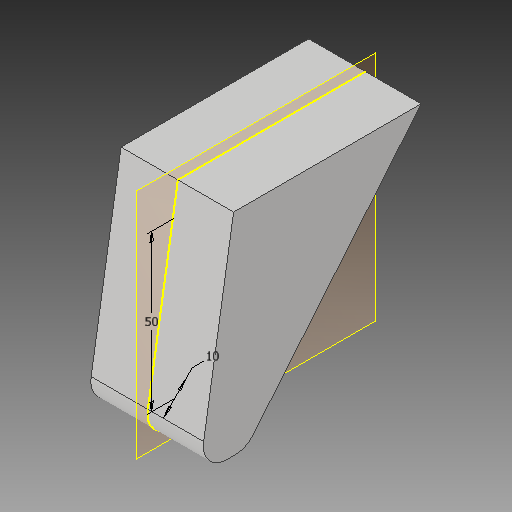
# Autodesk Inventor part: Part_MetalLeg
Saved by Autodesk Inventor 2019 (Build 230136000, 136)
## iProperties
Created: 2019-04-26
Part Number: Part_MetalLeg
Material: 일반
Document SubType Name: Modeling
Designer: hinmo
Density: 1 g/cm^3
Appearance: 기본값
Author: hinmo
Autodesk Inventor part; units mm, degrees
ref_plane "YZ Plane" through (0, 0, 0) normal (1, 0, 0) x (0, 1, 0)
ref_plane "XZ Plane" through (0, 0, 0) normal (0, 1, 0) x (-1, 0, 0)
ref_plane "XY Plane" through (0, 0, 0) normal (0, 0, 1) x (1, 0, 0)
sketch "스케치1" plane through (0, 0, 0) normal (1, 0, 0) x (0, 1, 0)
  line L0 (-33.75, 41) -> (33.75, 41)
  line L1 (33.75, 41) -> (33.75, -41)
  line L2 (33.75, -41) -> (-33.75, -41)
  line L3 (-33.75, 29.5228) -> (-33.75, 32.1788)
  line L4 (-33.75, 41) -> (33.75, -41) construction
  line L5 (33.75, 41) -> (-33.75, -41) construction
  line L6 (33.75, 41) -> (33.75, 35)
  line L7 (33.75, 0) -> (33.75, 30)
  line L8 (33.75, 30) -> (-25.0437, 39.5812)
  line L9 (33.75, 0) -> (33.75, -30)
  line L10 (-31.0388, 23.7507) -> (33.75, -30)
  arc A0 (-33.75, 29.5228) -> (-31.0388, 23.7507) centre (-26.25, 29.5228) ccw
  arc A1 (-25.0437, 39.5812) -> (-33.75, 32.1788) centre (-26.25, 32.1788) ccw
  point P0 (0, 0)
  point P1 (-33.75, 26)
  dimension "d3" = 67.5
  dimension "d4" = 82
  dimension "d6" = 30
  dimension "d7" = 30
  dimension "d9" = 15
  dimension "d10" = 7.5
  constraints: 22 end point, 7 point on line, 4 point on circle, 4 tangent, 3 midpoint, 2 centre point, 2 parallel, 1 equal radius, 1 horizontal, 1 perpendicular
  measures "d3" distance of L1.end L2.end
  measures "d4" distance of L0.end L1.end
  measures "d6" distance of L7.start L7.end
  measures "d7" distance of L7.start L9.end
  measures "d9" distance of point (-33.75, 26) L0.start
  measures "d10" radius of A0
extrude "돌출1" add sketch "스케치1" along normal blind 36
ref_plane "작업 평면1" through (18, 0, 0) normal (1, 0, 0) x (0, 0, -1)
sketch "스케치2" plane through (18, 0, 0) normal (1, 0, 0) x (0, 0, -1)
  line L0 (-30, 33.75) -> (-39.5812, -25.0437) projected
  arc A0 (-39.5812, -25.0437) -> (-32.1788, -33.75) centre (-32.1788, -26.25) ccw projected
  line L1 (-32.1788, -33.75) -> (-29.5228, -33.75) projected
  arc A1 (-29.5228, -33.75) -> (-23.7507, -31.0388) centre (-29.5228, -26.25) ccw projected
  line L2 (-23.7507, -31.0388) -> (30, 33.75) projected
  line L3 (30, 33.75) -> (-30, 33.75) projected
  line L4 (30, 33.75) -> (-30, 33.75) projected
  line L5 (-30, 33.75) -> (-39.5812, -25.0437) projected
  circle A2 centre (-30.8508, -26.4664) radius 5
  line L6 (-30.8508, -26.4664) -> (-30.8508, 23.5336)
  line L7 (-30.8508, 23.5336) -> (21.5242, 23.5336)
  line L8 (-23.7507, -31.0388) -> (30, 33.75) projected
  point P0 (0, 0)
  dimension "d14" = 10
  dimension "d15" = 50
  constraints: 4 end point, 1 centre point, 1 horizontal, 1 point on line, 1 vertical
  measures "d14" diameter of A2
  measures "d15" distance of L6.start L6.end
